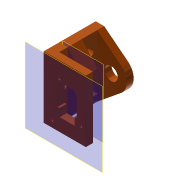
# Autodesk Inventor part: 30_cellSTORM_fiberbase_base_v3
Saved by Autodesk Inventor 2019.4 (Build 234330000, 330)
## iProperties
Created: 2021-07-02
Part Number: 30_cellSTORM_fiberbase_base_v3
Material: Generic
Document SubType Name: Modeling
Designer: diederichbenedict
Density: 1 g/cm^3
Appearance: Smooth - Light Orange
Mass: 18.3475 g
Surface Area: 86.0517 cm^2
Volume: 18.3475 cm^3
Author: diederichbenedict
Autodesk Inventor part; units mm, degrees
note: some values were not read from the file. Chosen so that the rebuilt part matches the saved one: sketch regions of "Extrusion3".
ref_plane "YZ Plane" through (0, 0, 0) normal (1, 0, 0) x (0, 1, 0)
ref_plane "XZ Plane" through (0, 0, 0) normal (0, 1, 0) x (-1, 0, 0)
ref_plane "Work Plane1" through (29.8677, -69.0107, 8.183) normal (0, 0, -1) x (-1, 0, 0)
sketch "Sketch1" plane through (29.8677, -69.0107, 8.183) normal (0, 0, -1) x (-1, 0, 0)
  line L0 (2.603, -2) -> (2.603, -17.5) projected
  line L1 (2.603, -17.5) -> (-10.897, -17.5) projected
  line L2 (-10.897, -17.5) -> (-10.897, -2) projected
  line L3 (-10.897, -2) -> (2.603, -2) projected
  circle A0 centre (6.603, -27.5) radius 1 projected
  circle A1 centre (-13.897, -21) radius 1 projected
  circle A2 centre (1.603, 0.5) radius 1 projected
  arc A3 (9.303, -26.8555) -> (8.303, -25.8555) centre (8.303, -26.8555) ccw projected
  line L4 (8.303, -25.8555) -> (5.5653, -25.8555) projected
  arc A4 (4.5653, -24.8555) -> (5.5653, -25.8555) centre (5.5653, -24.8555) ccw projected
  line L5 (4.5653, -24.8555) -> (4.5653, 2) projected
  arc A5 (4.5653, 2) -> (3.5653, 3) centre (3.5653, 2) ccw projected
  line L6 (3.5653, 3) -> (1, 3) projected
  arc A6 (1, 3) -> (0, 2) centre (1, 2) ccw projected
  line L7 (0, 2) -> (0, 1) projected
  arc A7 (-1, 0) -> (0, 1) centre (-1, 1) ccw projected
  line L8 (-1, 0) -> (-12.5347, 0) projected
  line L9 (-12.5347, 0) -> (-12.5347, -18.4723) projected
  arc A8 (-13.5347, -19.4723) -> (-12.5347, -18.4723) centre (-13.5347, -18.4723) ccw projected
  line L10 (-13.5347, -19.4723) -> (-15.397, -19.4723) projected
  arc A9 (-15.397, -19.4723) -> (-16.397, -20.4723) centre (-15.397, -20.4723) ccw projected
  line L11 (-16.397, -20.4723) -> (-16.397, -30) projected
  line L12 (-16.397, -30) -> (9.303, -30) projected
  line L13 (9.303, -30) -> (9.303, -26.8555) projected
  line L14 (-17.397, 11.7453) -> (12.5653, 11.7453)
  line L15 (12.5653, 11.7453) -> (12.5653, -32.2547)
  line L16 (12.5653, -32.2547) -> (-17.397, -32.2547)
  line L17 (-17.397, -32.2547) -> (-17.397, 11.7453)
  line L18 (1.2141, -1.4589) -> (-9.519, -1.4589)
  line L19 (-9.519, -1.4589) -> (-9.519, -23.1404)
  line L20 (-9.519, -23.1404) -> (1.2141, -23.1404)
  line L21 (1.2141, -23.1404) -> (1.2141, -1.4589)
  ellipse E0 centre (-3.397, -10.2547) end of major axis (-6.4323, -10.2547) minor radius 3.0277 projected
  point P0 (29.8677, 69.0107)
  dimension "d0" = 8
  dimension "d1" = 1
  dimension "d13" = 22
  dimension "d14" = 22
  constraints: 16 end point, 4 parallel, 2 horizontal, 2 perpendicular, 1 other
  measures "d0" distance between parallel lines of L15 L5
  measures "d1" distance between parallel lines of L11 L17
  measures "d13" distance from line of L14 point (-3.397, -10.255)
  measures "d14" distance from line of L16 point (-3.397, -10.255)
extrude "Extrusion1" add sketch "Sketch1" along normal blind 5 contours L13 L12 L11 A9 L10 A8 L9 L8 A7 L7 A6 L6 A5 L5 A4 L4 A3 | L14 L15 L16 L17
sketch "Sketch2" plane through (29.8677, -69.0107, 3.183) normal (0, 0, -1) x (-1, 0, 0)
  line L0 (12.5653, 11.7453) -> (-17.397, 11.7453) projected
  line L1 (-17.397, 11.7453) -> (-17.397, -32.2547) projected
  line L2 (-17.397, -32.2547) -> (12.5653, -32.2547) projected
  line L3 (12.5653, -32.2547) -> (12.5653, 11.7453) projected
  circle A0 centre (6.603, -27.5) radius 1 projected
  circle A1 centre (-13.897, -21) radius 1 projected
  circle A2 centre (1.603, 0.5) radius 1 projected
  line L4 (1.2141, -17.5) -> (1.2141, -23.1404) projected
  line L5 (1.2141, -23.1404) -> (-9.519, -23.1404) projected
  line L6 (-9.519, -23.1404) -> (-9.519, -17.5) projected
  line L7 (-9.519, -17.5) -> (-10.897, -17.5) projected
  line L8 (-10.897, -17.5) -> (-10.897, -2) projected
  line L9 (-10.897, -2) -> (-9.519, -2) projected
  line L10 (-9.519, -2) -> (-9.519, -1.4589) projected
  line L11 (-9.519, -1.4589) -> (1.2141, -1.4589) projected
  line L12 (1.2141, -1.4589) -> (1.2141, -2) projected
  line L13 (1.2141, -2) -> (2.603, -2) projected
  line L14 (2.603, -2) -> (2.603, -17.5) projected
  line L15 (2.603, -17.5) -> (1.2141, -17.5) projected
  line L16 (-17.397, 11.7453) -> (12.5653, 11.7453) projected
  line L17 (12.5653, -32.2547) -> (-17.397, -32.2547) projected
  line L18 (12.5653, 11.7453) -> (6.5653, 11.7453)
  line L19 (6.5653, 11.7453) -> (6.5653, -32.2547)
  line L20 (6.5653, -32.2547) -> (12.5653, -32.2547)
  line L21 (12.5653, -32.2547) -> (12.5653, 11.7453)
  point P0 (29.8677, 69.0107)
  dimension "d6" = 6
  constraints: 8 end point, 2 parallel, 1 horizontal, 1 perpendicular, 1 point on line
  measures "d6" distance of L20.end L19.end
extrude "Extrusion2" add sketch "Sketch2" along normal blind 32 contours L3 L2 L19 A0 L0 | A0 L19 picked at (6.9324, -27.235)
sketch "Sketch3" plane through (29.8677, -69.0107, -28.817) normal (0, 0, -1) x (-1, 0, 0)
  circle A0 centre (-3.397, -10) radius 4.445 projected
  circle A1 centre (-3.397, -10) radius 4.645
  line L0 (12.5653, 11.7453) -> (12.5653, -32.2547) projected
  line L1 (12.5653, -32.2547) -> (12.5653, 11.7453) projected
  line L2 (12.5653, 11.7453) -> (6.5653, 11.7453) projected
  line L3 (6.5653, 11.7453) -> (6.5653, -32.2547) projected
  line L4 (6.5653, -32.2547) -> (12.5653, -32.2547) projected
  line L5 (12.5653, -32.2547) -> (12.5653, 11.7453) projected
  line L6 (6.5653, 11.7453) -> (-17.397, 11.7453) projected
  line L7 (-9.2429, -0.682) -> (6.5653, 11.7453)
  line L8 (-9.5834, -19.0955) -> (6.5653, -32.2547)
  line L9 (6.5653, 11.7453) -> (6.5653, -5.3362)
  line L10 (6.5653, -14.6638) -> (6.5653, -32.2547)
  arc A2 (-9.2429, -0.682) -> (-9.5834, -19.0955) centre (-3.397, -10) ccw
  arc A3 (6.5653, -14.6638) -> (6.5653, -5.3362) centre (-3.397, -10) ccw
  point P0 (29.8677, 69.0107)
  dimension "d9" = 0.2
  constraints: 8 end point, 4 point on circle, 3 centre point, 2 perpendicular, 1 coincident
  measures "d9" radial gap between concentric circles of A0 A1
ref_plane "Work Plane2" through (26.9102, -85.3653, -23.8679) normal (0, 0, -1) x (0, 1, 0)
extrude "Extrusion3" add sketch "Sketch3" against normal up to surface (4.9491 mm away) contours L0 L4 L3 A3 L2 | L3 L8 A2 L7 | A3 L3
ref_plane "Work Plane3" through (29.8677, -69.0107, -2.817) normal (0, 0, -1) x (-1, 0, 0)
sketch "Sketch4" plane through (29.8677, -69.0107, -2.817) normal (0, 0, -1) x (-1, 0, 0)
  circle A0 centre (-3.397, -10) radius 6.35 projected
  line L0 (6.5653, -32.2547) -> (6.5653, 11.7453) projected
  line L1 (6.5653, -32.2547) -> (-4.8237, -20.0055)
  line L2 (-4.8237, -20.0055) -> (-4.8237, -16.1877)
  line L3 (12.5653, -32.2547) -> (-17.397, -32.2547) projected
  line L4 (6.5653, 11.7453) -> (-4.8237, -0.7453)
  line L5 (-4.8237, -0.7453) -> (-4.8237, -3.8123)
  point P0 (29.8677, 69.0107)
  constraints: 8 end point, 2 point on circle, 2 point on line, 1 perpendicular
extrude "Extrusion4" add sketch "Sketch4" along normal blind 10 contours A0 L5 L4 L0 L1 L2
sketch "Sketch5" plane through (23.3024, -101.2655, -23.8679) normal (1, 0, 0) x (0, 0, -1)
  line L0 (-21.0509, 0) -> (-21.0509, 44) projected
  line L1 (-27.0509, 44) -> (-21.0509, 44) projected
  line L2 (-27.0509, 0) -> (-27.0509, 3.7554) projected
  line L3 (-27.0509, 0) -> (-21.0509, 0) projected
  line L4 (-11.0509, 44) -> (-11.0509, 0) projected
  line L5 (-11.0509, 0) -> (0, 0) projected
  line L6 (-11.0509, 44) -> (0, 44) projected
  line L7 (-5.3231, 32.8665) -> (-5.3231, 11.3659)
  line L8 (-5.3231, 11.3659) -> (-23.9432, 22.1162)
  line L9 (-23.9432, 22.1162) -> (-5.3231, 32.8665)
  circle A0 centre (-23.9432, 22.1162) radius 3
  circle A1 centre (-5.3231, 32.8665) radius 3
  circle A2 centre (-5.3231, 11.3659) radius 3
  line L10 (-27.0509, 0) -> (-21.0509, 0) projected
  line L11 (-27.0509, 44) -> (-21.0509, 44) projected
  line L12 (-21.0509, 0) -> (-21.0509, 44) projected
  line L13 (-27.0509, 5.754) -> (-27.0509, 44) projected
  line L14 (-27.0509, 5.754) -> (-27.0509, 3.7554) projected
  line L15 (-27.0509, 0) -> (-27.0509, 3.7554) projected
  line L16 (-27.0509, 5.754) -> (-27.0509, 44) projected
  line L17 (-27.0509, 5.754) -> (-27.0509, 3.7554) projected
  line L18 (0, 0) -> (0, 44) projected
  point P0 (-23.8679, 101.2655)
  point P1 (-11.5298, 22.1162)
  dimension "d18" = 0
  dimension "d19" = 6
  dimension "d20" = 6
  dimension "d21" = 6
  constraints: 6 end point, 3 centre point, 3 coincident, 7 other
  measures "d18" angle of L4 L7
  measures "d19" diameter of A0
  measures "d20" diameter of A1
  measures "d21" diameter of A2
extrude "Extrusion5" cut sketch "Sketch5" against normal blind 10 contours A0 L8 L9 L0 | L0 A0 | A0 L9 L8 | A2 L7 L8 | L8 L7 A2 | A1 L7 L9 | L9 L7 A1
body "Solid1"
